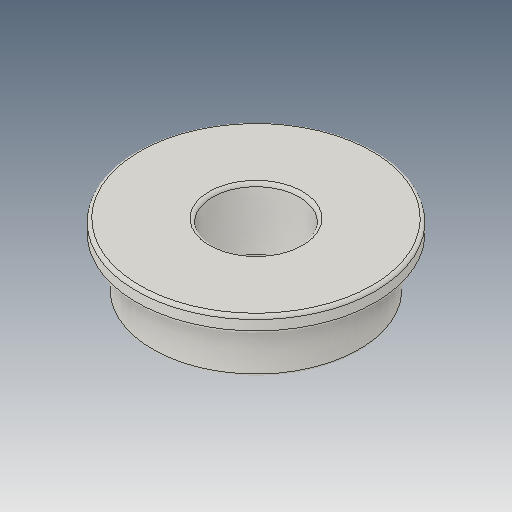
# Autodesk Inventor part: p8-19flange
Saved by Autodesk Inventor 2019.4 (Build 234330000, 330)
## iProperties
Created: 2019-06-11
Part Number: p8-19flange
Material: 鋼 AISI 1006 85 HR
Document SubType Name: Modeling
Designer: AzLIer
Density: 7.872 g/cm^3
Appearance: 鋼
Mass: 12.1205 g
Surface Area: 11.5081 cm^2
Volume: 1.5397 cm^3
Author: AzLIer
Autodesk Inventor part; units mm, degrees
ref_plane "YZ Plane" through (0, 0, 0) normal (1, 0, 0) x (0, 1, 0)
ref_plane "XZ Plane" through (0, 0, 0) normal (0, 1, 0) x (-1, 0, 0)
ref_plane "XY Plane" through (0, 0, 0) normal (0, 0, 1) x (1, 0, 0)
sketch "スケッチ1" plane through (0, 0, 0) normal (0, 1, 0) x (-1, 0, 0)
  circle A0 centre (0, 0) radius 4
  circle A1 centre (0, 0) radius 9.5
  dimension "d0" = 8
  dimension "d1" = 19
  constraints: 2 centre point, 2 coincident
  measures "d0" diameter of A0
  measures "d1" diameter of A1
extrude "押し出し1" add sketch "スケッチ1" along normal blind 6
sketch "スケッチ2" plane through (0, 6, 0) normal (0, 1, 0) x (1, 0, 0)
  circle A0 centre (0, 0) radius 11
  circle A1 centre (0, 0) radius 9.5 projected
  dimension "d4" = 22
  constraints: 1 centre point, 1 coincident
  measures "d4" diameter of A0
extrude "押し出し2" add sketch "スケッチ2" against normal blind 1.5
fillet "フィレット1" radius 0.3 5 edges at (-11, 6, 0) (-11, 4.5, 0) (9.5, 0, 0) (4, 6, 0) (4, 0, 0)
